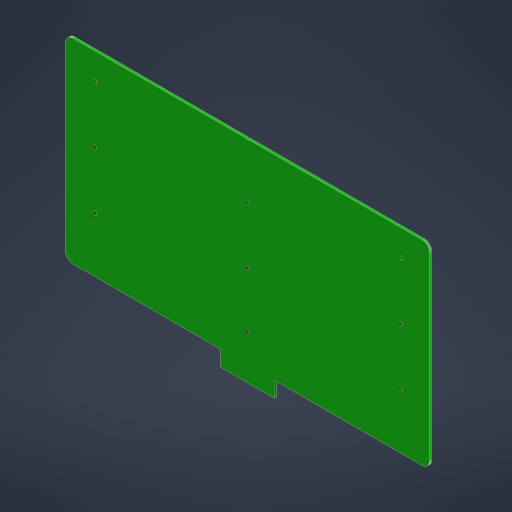
# Autodesk Inventor part: Platine_unten
Saved by Autodesk Inventor 2024.3 (Build 283343010, 343A)
## iProperties
Created: 2025-05-08
Part Number: Platine_unten
Material: Generisch
Document SubType Name: Modeling
Designer: David
Density: 1 g/cm^3
Appearance: Glatt - Schwarz
Author: David
Autodesk Inventor part; units mm, degrees
ref_plane "YZ Plane" through (0, 0, 0) normal (1, 0, 0) x (0, 1, 0)
ref_plane "XZ Plane" through (0, 0, 0) normal (0, 1, 0) x (-1, 0, 0)
ref_plane "XY Plane" through (0, 0, 0) normal (0, 0, 1) x (1, 0, 0)
sketch "Skizze1" plane through (0, 0, 0) normal (0, 1, 0) x (-1, 0, 0)
  line L0 (149.0026, -15.3777) -> (148.6057, -15.2961)
  line L1 (148.6057, -15.2961) -> (148.2026, -15.2551)
  line L2 (148.2026, -15.2551) -> (147.7974, -15.2551)
  line L3 (147.7974, -15.2551) -> (147.3943, -15.2961)
  line L4 (147.3943, -15.2961) -> (146.9974, -15.3777)
  line L5 (146.9974, -15.3777) -> (146.6108, -15.499)
  line L6 (146.6108, -15.499) -> (146.2384, -15.6588)
  line L7 (146.2384, -15.6588) -> (145.8841, -15.8554)
  line L8 (145.8841, -15.8554) -> (145.5516, -16.0869)
  line L9 (145.5516, -16.0869) -> (145.2441, -16.3508)
  line L10 (145.2441, -16.3508) -> (144.965, -16.6445)
  line L11 (144.965, -16.6445) -> (144.7169, -16.9649)
  line L12 (144.7169, -16.9649) -> (144.5026, -17.3088)
  line L13 (144.5026, -17.3088) -> (144.3242, -17.6726)
  line L14 (144.3242, -17.6726) -> (144.1834, -18.0525)
  line L15 (144.1834, -18.0525) -> (144.0819, -18.4448)
  line L16 (144.0819, -18.4448) -> (144.0205, -18.8453)
  line L17 (144.0205, -18.8453) -> (144, -19.25)
  line L18 (144, -19.25) -> (144, -20.5)
  line L19 (144, -20.5) -> (152, -20.5)
  line L20 (152, -20.5) -> (152, -19.25)
  line L21 (152, -19.25) -> (151.9795, -18.8453)
  line L22 (151.9795, -18.8453) -> (151.9181, -18.4448)
  line L23 (151.9181, -18.4448) -> (151.8166, -18.0525)
  line L24 (151.8166, -18.0525) -> (151.6758, -17.6726)
  line L25 (151.6758, -17.6726) -> (151.4974, -17.3088)
  line L26 (151.4974, -17.3088) -> (151.2831, -16.9649)
  line L27 (151.2831, -16.9649) -> (151.035, -16.6445)
  line L28 (151.035, -16.6445) -> (150.7559, -16.3508)
  line L29 (150.7559, -16.3508) -> (150.4484, -16.0869)
  line L30 (150.4484, -16.0869) -> (150.1159, -15.8554)
  line L31 (150.1159, -15.8554) -> (149.7616, -15.6588)
  line L32 (149.7616, -15.6588) -> (149.3892, -15.499)
  line L33 (149.3892, -15.499) -> (149.0026, -15.3777)
  line L34 (144, -20.5) -> (25, -20.5)
  line L35 (25, -20.5) -> (24.5642, -20.519)
  line L36 (24.5642, -20.519) -> (24.1318, -20.576)
  line L37 (24.1318, -20.576) -> (23.7059, -20.6704)
  line L38 (23.7059, -20.6704) -> (23.2899, -20.8015)
  line L39 (23.2899, -20.8015) -> (22.8869, -20.9685)
  line L40 (22.8869, -20.9685) -> (22.5, -21.1699)
  line L41 (22.5, -21.1699) -> (22.1321, -21.4042)
  line L42 (22.1321, -21.4042) -> (21.7861, -21.6698)
  line L43 (21.7861, -21.6698) -> (21.4645, -21.9645)
  line L44 (21.4645, -21.9645) -> (21.1698, -22.2861)
  line L45 (21.1698, -22.2861) -> (20.9042, -22.6321)
  line L46 (20.9042, -22.6321) -> (20.6699, -23)
  line L47 (20.6699, -23) -> (20.4685, -23.3869)
  line L48 (20.4685, -23.3869) -> (20.3015, -23.7899)
  line L49 (20.3015, -23.7899) -> (20.1704, -24.2059)
  line L50 (20.1704, -24.2059) -> (20.076, -24.6318)
  line L51 (20.076, -24.6318) -> (20.019, -25.0642)
  line L52 (20.019, -25.0642) -> (20, -25.5)
  line L53 (20, -25.5) -> (20, -153)
  line L54 (20, -153) -> (20.019, -153.4358)
  line L55 (20.019, -153.4358) -> (20.076, -153.8682)
  line L56 (20.076, -153.8682) -> (20.1704, -154.2941)
  line L57 (20.1704, -154.2941) -> (20.3015, -154.7101)
  line L58 (20.3015, -154.7101) -> (20.4685, -155.1131)
  line L59 (20.4685, -155.1131) -> (20.6699, -155.5)
  line L60 (20.6699, -155.5) -> (20.9042, -155.8679)
  line L61 (20.9042, -155.8679) -> (21.1698, -156.2139)
  line L62 (21.1698, -156.2139) -> (21.4645, -156.5355)
  line L63 (21.4645, -156.5355) -> (21.7861, -156.8302)
  line L64 (21.7861, -156.8302) -> (22.1321, -157.0958)
  line L65 (22.1321, -157.0958) -> (22.5, -157.3301)
  line L66 (22.5, -157.3301) -> (22.8869, -157.5315)
  line L67 (22.8869, -157.5315) -> (23.2899, -157.6985)
  line L68 (23.2899, -157.6985) -> (23.7059, -157.8296)
  line L69 (23.7059, -157.8296) -> (24.1318, -157.924)
  line L70 (24.1318, -157.924) -> (24.5642, -157.981)
  line L71 (24.5642, -157.981) -> (25, -158)
  line L72 (25, -158) -> (129, -158)
  line L73 (129, -158) -> (129, -169)
  line L74 (129, -169) -> (167, -169)
  line L75 (167, -169) -> (167, -158)
  line L76 (167, -158) -> (271, -158)
  line L77 (271, -158) -> (271.4358, -157.981)
  line L78 (271.4358, -157.981) -> (271.8682, -157.924)
  line L79 (271.8682, -157.924) -> (272.2941, -157.8296)
  line L80 (272.2941, -157.8296) -> (272.7101, -157.6985)
  line L81 (272.7101, -157.6985) -> (273.1131, -157.5315)
  line L82 (273.1131, -157.5315) -> (273.5, -157.3301)
  line L83 (273.5, -157.3301) -> (273.8679, -157.0958)
  line L84 (273.8679, -157.0958) -> (274.2139, -156.8302)
  line L85 (274.2139, -156.8302) -> (274.5355, -156.5355)
  line L86 (274.5355, -156.5355) -> (274.8302, -156.2139)
  line L87 (274.8302, -156.2139) -> (275.0958, -155.8679)
  line L88 (275.0958, -155.8679) -> (275.3301, -155.5)
  line L89 (275.3301, -155.5) -> (275.5315, -155.1131)
  line L90 (275.5315, -155.1131) -> (275.6985, -154.7101)
  line L91 (275.6985, -154.7101) -> (275.8296, -154.2941)
  line L92 (275.8296, -154.2941) -> (275.924, -153.8682)
  line L93 (275.924, -153.8682) -> (275.981, -153.4358)
  line L94 (275.981, -153.4358) -> (276, -153)
  line L95 (276, -153) -> (276, -25.5)
  line L96 (276, -25.5) -> (275.981, -25.0642)
  line L97 (275.981, -25.0642) -> (275.924, -24.6318)
  line L98 (275.924, -24.6318) -> (275.8296, -24.2059)
  line L99 (275.8296, -24.2059) -> (275.6985, -23.7899)
  line L100 (275.6985, -23.7899) -> (275.5315, -23.3869)
  line L101 (275.5315, -23.3869) -> (275.3301, -23)
  line L102 (275.3301, -23) -> (275.0958, -22.6321)
  line L103 (275.0958, -22.6321) -> (274.8302, -22.2861)
  line L104 (274.8302, -22.2861) -> (274.5355, -21.9645)
  line L105 (274.5355, -21.9645) -> (274.2139, -21.6698)
  line L106 (274.2139, -21.6698) -> (273.8679, -21.4042)
  line L107 (273.8679, -21.4042) -> (273.5, -21.1699)
  line L108 (273.5, -21.1699) -> (273.1131, -20.9685)
  line L109 (273.1131, -20.9685) -> (272.7101, -20.8015)
  line L110 (272.7101, -20.8015) -> (272.2941, -20.6704)
  line L111 (272.2941, -20.6704) -> (271.8682, -20.576)
  line L112 (271.8682, -20.576) -> (271.4358, -20.519)
  line L113 (271.4358, -20.519) -> (271, -20.5)
  line L114 (271, -20.5) -> (152, -20.5)
  line L115 (152, -20.5) -> (144, -20.5)
  line L116 (129, -169) -> (167, -169)
  line L117 (167, -169) -> (167, -158)
  line L118 (167, -158) -> (271, -158)
  line L119 (271, -158) -> (271.4358, -157.981)
  line L120 (271.4358, -157.981) -> (271.8682, -157.924)
  line L121 (271.8682, -157.924) -> (272.2941, -157.8296)
  line L122 (272.2941, -157.8296) -> (272.7101, -157.6985)
  line L123 (272.7101, -157.6985) -> (273.1131, -157.5315)
  line L124 (273.1131, -157.5315) -> (273.5, -157.3301)
  line L125 (273.5, -157.3301) -> (273.8679, -157.0958)
  line L126 (273.8679, -157.0958) -> (274.2139, -156.8302)
  line L127 (274.2139, -156.8302) -> (274.5355, -156.5355)
  line L128 (274.5355, -156.5355) -> (274.8302, -156.2139)
  line L129 (274.8302, -156.2139) -> (275.0958, -155.8679)
  line L130 (275.0958, -155.8679) -> (275.3301, -155.5)
  line L131 (275.3301, -155.5) -> (275.5315, -155.1131)
  line L132 (275.5315, -155.1131) -> (275.6985, -154.7101)
  line L133 (275.6985, -154.7101) -> (275.8296, -154.2941)
  line L134 (275.8296, -154.2941) -> (275.924, -153.8682)
  line L135 (275.924, -153.8682) -> (275.981, -153.4358)
  line L136 (275.981, -153.4358) -> (276, -153)
  line L137 (276, -153) -> (276, -25.5)
  line L138 (276, -25.5) -> (275.981, -25.0642)
  line L139 (275.981, -25.0642) -> (275.924, -24.6318)
  line L140 (275.924, -24.6318) -> (275.8296, -24.2059)
  line L141 (275.8296, -24.2059) -> (275.6985, -23.7899)
  line L142 (275.6985, -23.7899) -> (275.5315, -23.3869)
  line L143 (275.5315, -23.3869) -> (275.3301, -23)
  line L144 (275.3301, -23) -> (275.0958, -22.6321)
  line L145 (275.0958, -22.6321) -> (274.8302, -22.2861)
  line L146 (274.8302, -22.2861) -> (274.5355, -21.9645)
  line L147 (274.5355, -21.9645) -> (274.2139, -21.6698)
  line L148 (274.2139, -21.6698) -> (273.8679, -21.4042)
  line L149 (273.8679, -21.4042) -> (273.5, -21.1699)
  line L150 (273.5, -21.1699) -> (273.1131, -20.9685)
  line L151 (273.1131, -20.9685) -> (272.7101, -20.8015)
  line L152 (272.7101, -20.8015) -> (272.2941, -20.6704)
  line L153 (272.2941, -20.6704) -> (271.8682, -20.576)
  line L154 (271.8682, -20.576) -> (271.4358, -20.519)
  line L155 (271.4358, -20.519) -> (271, -20.5)
  line L156 (271, -20.5) -> (152, -20.5)
  line L157 (152, -20.5) -> (152, -19.25)
  line L158 (152, -19.25) -> (151.9795, -18.8453)
  line L159 (151.9795, -18.8453) -> (151.9181, -18.4448)
  line L160 (151.9181, -18.4448) -> (151.8166, -18.0525)
  line L161 (151.8166, -18.0525) -> (151.6758, -17.6726)
  line L162 (151.6758, -17.6726) -> (151.4974, -17.3088)
  line L163 (151.4974, -17.3088) -> (151.2831, -16.9649)
  line L164 (151.2831, -16.9649) -> (151.035, -16.6445)
  line L165 (151.035, -16.6445) -> (150.7559, -16.3508)
  line L166 (150.7559, -16.3508) -> (150.4484, -16.0869)
  line L167 (150.4484, -16.0869) -> (150.1159, -15.8554)
  line L168 (150.1159, -15.8554) -> (149.7616, -15.6588)
  line L169 (149.7616, -15.6588) -> (149.3892, -15.499)
  line L170 (149.3892, -15.499) -> (149.0026, -15.3777)
  line L171 (149.0026, -15.3777) -> (148.6057, -15.2961)
  line L172 (148.6057, -15.2961) -> (148.2026, -15.2551)
  line L173 (148.2026, -15.2551) -> (147.7974, -15.2551)
  line L174 (147.7974, -15.2551) -> (147.3943, -15.2961)
  line L175 (147.3943, -15.2961) -> (146.9974, -15.3777)
  line L176 (146.9974, -15.3777) -> (146.6108, -15.499)
  line L177 (146.6108, -15.499) -> (146.2384, -15.6588)
  line L178 (146.2384, -15.6588) -> (145.8841, -15.8554)
  line L179 (145.8841, -15.8554) -> (145.5516, -16.0869)
  line L180 (145.5516, -16.0869) -> (145.2441, -16.3508)
  line L181 (145.2441, -16.3508) -> (144.965, -16.6445)
  line L182 (144.965, -16.6445) -> (144.7169, -16.9649)
  line L183 (144.7169, -16.9649) -> (144.5026, -17.3088)
  line L184 (144.5026, -17.3088) -> (144.3242, -17.6726)
  line L185 (144.3242, -17.6726) -> (144.1834, -18.0525)
  line L186 (144.1834, -18.0525) -> (144.0819, -18.4448)
  line L187 (144.0819, -18.4448) -> (144.0205, -18.8453)
  line L188 (144.0205, -18.8453) -> (144, -19.25)
  line L189 (144, -19.25) -> (144, -20.5)
  line L190 (144, -20.5) -> (25, -20.5)
  line L191 (25, -20.5) -> (24.5642, -20.519)
  line L192 (24.5642, -20.519) -> (24.1318, -20.576)
  line L193 (24.1318, -20.576) -> (23.7059, -20.6704)
  line L194 (23.7059, -20.6704) -> (23.2899, -20.8015)
  line L195 (23.2899, -20.8015) -> (22.8869, -20.9685)
  line L196 (22.8869, -20.9685) -> (22.5, -21.1699)
  line L197 (22.5, -21.1699) -> (22.1321, -21.4042)
  line L198 (22.1321, -21.4042) -> (21.7861, -21.6698)
  line L199 (21.7861, -21.6698) -> (21.4645, -21.9645)
  line L200 (21.4645, -21.9645) -> (21.1698, -22.2861)
  line L201 (21.1698, -22.2861) -> (20.9042, -22.6321)
  line L202 (20.9042, -22.6321) -> (20.6699, -23)
  line L203 (20.6699, -23) -> (20.4685, -23.3869)
  line L204 (20.4685, -23.3869) -> (20.3015, -23.7899)
  line L205 (20.3015, -23.7899) -> (20.1704, -24.2059)
  line L206 (20.1704, -24.2059) -> (20.076, -24.6318)
  line L207 (20.076, -24.6318) -> (20.019, -25.0642)
  line L208 (20.019, -25.0642) -> (20, -25.5)
  line L209 (20, -25.5) -> (20, -153)
  line L210 (20, -153) -> (20.019, -153.4358)
  line L211 (20.019, -153.4358) -> (20.076, -153.8682)
  line L212 (20.076, -153.8682) -> (20.1704, -154.2941)
  line L213 (20.1704, -154.2941) -> (20.3015, -154.7101)
  line L214 (20.3015, -154.7101) -> (20.4685, -155.1131)
  line L215 (20.4685, -155.1131) -> (20.6699, -155.5)
  line L216 (20.6699, -155.5) -> (20.9042, -155.8679)
  line L217 (20.9042, -155.8679) -> (21.1698, -156.2139)
  line L218 (21.1698, -156.2139) -> (21.4645, -156.5355)
  line L219 (21.4645, -156.5355) -> (21.7861, -156.8302)
  line L220 (21.7861, -156.8302) -> (22.1321, -157.0958)
  line L221 (22.1321, -157.0958) -> (22.5, -157.3301)
  line L222 (22.5, -157.3301) -> (22.8869, -157.5315)
  line L223 (22.8869, -157.5315) -> (23.2899, -157.6985)
  line L224 (23.2899, -157.6985) -> (23.7059, -157.8296)
  line L225 (23.7059, -157.8296) -> (24.1318, -157.924)
  line L226 (24.1318, -157.924) -> (24.5642, -157.981)
  line L227 (24.5642, -157.981) -> (25, -158)
  line L228 (25, -158) -> (129, -158)
  line L229 (129, -158) -> (129, -169)
  line L230 (137.25, -162.4) -> (137.25, -165.9)
  line L231 (137.25, -165.9) -> (158.75, -165.9)
  line L232 (158.75, -165.9) -> (137.25, -165.9)
  line L233 (137.25, -165.9) -> (158.75, -165.9)
  line L234 (158.75, -165.9) -> (158.75, -162.4)
  line L235 (158.75, -162.4) -> (137.25, -162.4)
  line L236 (137.75, -162.9) -> (140.25, -162.9)
  line L237 (140.25, -162.9) -> (140.25, -165.4)
  line L238 (140.25, -165.4) -> (137.75, -165.4)
  line L239 (137.75, -165.4) -> (137.75, -162.9)
  line L240 (140.75, -162.9) -> (143.25, -162.9)
  line L241 (143.25, -162.9) -> (143.25, -165.4)
  line L242 (143.25, -165.4) -> (140.75, -165.4)
  line L243 (140.75, -165.4) -> (140.75, -162.9)
  line L244 (143.75, -162.9) -> (146.25, -162.9)
  line L245 (146.25, -162.9) -> (146.25, -165.4)
  line L246 (146.25, -165.4) -> (143.75, -165.4)
  line L247 (143.75, -165.4) -> (143.75, -162.9)
  line L248 (146.75, -162.9) -> (149.25, -162.9)
  line L249 (149.25, -162.9) -> (149.25, -165.4)
  line L250 (149.25, -165.4) -> (146.75, -165.4)
  line L251 (146.75, -165.4) -> (146.75, -162.9)
  line L252 (149.75, -162.9) -> (152.25, -162.9)
  line L253 (152.25, -162.9) -> (152.25, -165.4)
  line L254 (152.25, -165.4) -> (149.75, -165.4)
  line L255 (149.75, -165.4) -> (149.75, -162.9)
  line L256 (152.75, -162.9) -> (155.25, -162.9)
  line L257 (155.25, -162.9) -> (155.25, -165.4)
  line L258 (155.25, -165.4) -> (152.75, -165.4)
  line L259 (152.75, -165.4) -> (152.75, -162.9)
  line L260 (155.75, -162.9) -> (158.25, -162.9)
  line L261 (158.25, -162.9) -> (158.25, -165.4)
  line L262 (158.25, -165.4) -> (155.75, -165.4)
  line L263 (155.75, -165.4) -> (155.75, -162.9)
  line L264 (129, -169) -> (129, -158)
  line L265 (129, -158) -> (25, -158)
  line L266 (25, -158) -> (24.5642, -157.981)
  line L267 (24.5642, -157.981) -> (24.1318, -157.924)
  line L268 (24.1318, -157.924) -> (23.7059, -157.8296)
  line L269 (23.7059, -157.8296) -> (23.2899, -157.6985)
  line L270 (23.2899, -157.6985) -> (22.8869, -157.5315)
  line L271 (22.8869, -157.5315) -> (22.5, -157.3301)
  line L272 (22.5, -157.3301) -> (22.1321, -157.0958)
  line L273 (22.1321, -157.0958) -> (21.7861, -156.8302)
  line L274 (21.7861, -156.8302) -> (21.4645, -156.5355)
  line L275 (21.4645, -156.5355) -> (21.1698, -156.2139)
  line L276 (21.1698, -156.2139) -> (20.9042, -155.8679)
  line L277 (20.9042, -155.8679) -> (20.6699, -155.5)
  line L278 (20.6699, -155.5) -> (20.4685, -155.1131)
  line L279 (20.4685, -155.1131) -> (20.3015, -154.7101)
  line L280 (20.3015, -154.7101) -> (20.1704, -154.2941)
  line L281 (20.1704, -154.2941) -> (20.076, -153.8682)
  line L282 (20.076, -153.8682) -> (20.019, -153.4358)
  line L283 (20.019, -153.4358) -> (20, -153)
  line L284 (20, -153) -> (20, -25.5)
  line L285 (20, -25.5) -> (20.019, -25.0642)
  line L286 (20.019, -25.0642) -> (20.076, -24.6318)
  line L287 (20.076, -24.6318) -> (20.1704, -24.2059)
  line L288 (20.1704, -24.2059) -> (20.3015, -23.7899)
  line L289 (20.3015, -23.7899) -> (20.4685, -23.3869)
  line L290 (20.4685, -23.3869) -> (20.6699, -23)
  line L291 (20.6699, -23) -> (20.9042, -22.6321)
  line L292 (20.9042, -22.6321) -> (21.1698, -22.2861)
  line L293 (21.1698, -22.2861) -> (21.4645, -21.9645)
  line L294 (21.4645, -21.9645) -> (21.7861, -21.6698)
  line L295 (21.7861, -21.6698) -> (22.1321, -21.4042)
  line L296 (22.1321, -21.4042) -> (22.5, -21.1699)
  line L297 (22.5, -21.1699) -> (22.8869, -20.9685)
  line L298 (22.8869, -20.9685) -> (23.2899, -20.8015)
  line L299 (23.2899, -20.8015) -> (23.7059, -20.6704)
  line L300 (23.7059, -20.6704) -> (24.1318, -20.576)
  line L301 (24.1318, -20.576) -> (24.5642, -20.519)
  line L302 (24.5642, -20.519) -> (25, -20.5)
  line L303 (25, -20.5) -> (144, -20.5)
  line L304 (144, -20.5) -> (144, -19.25)
  line L305 (144, -19.25) -> (144.0205, -18.8453)
  line L306 (144.0205, -18.8453) -> (144.0819, -18.4448)
  line L307 (144.0819, -18.4448) -> (144.1834, -18.0525)
  line L308 (144.1834, -18.0525) -> (144.3242, -17.6726)
  line L309 (144.3242, -17.6726) -> (144.5026, -17.3088)
  line L310 (144.5026, -17.3088) -> (144.7169, -16.9649)
  line L311 (144.7169, -16.9649) -> (144.965, -16.6445)
  line L312 (144.965, -16.6445) -> (145.2441, -16.3508)
  line L313 (145.2441, -16.3508) -> (145.5516, -16.0869)
  line L314 (145.5516, -16.0869) -> (145.8841, -15.8554)
  line L315 (145.8841, -15.8554) -> (146.2384, -15.6588)
  line L316 (146.2384, -15.6588) -> (146.6108, -15.499)
  line L317 (146.6108, -15.499) -> (146.9974, -15.3777)
  line L318 (146.9974, -15.3777) -> (147.3943, -15.2961)
  line L319 (147.3943, -15.2961) -> (147.7974, -15.2551)
  line L320 (147.7974, -15.2551) -> (148.2026, -15.2551)
  line L321 (148.2026, -15.2551) -> (148.6057, -15.2961)
  line L322 (148.6057, -15.2961) -> (149.0026, -15.3777)
  line L323 (149.0026, -15.3777) -> (149.3892, -15.499)
  line L324 (149.3892, -15.499) -> (149.7616, -15.6588)
  line L325 (149.7616, -15.6588) -> (150.1159, -15.8554)
  line L326 (150.1159, -15.8554) -> (150.4484, -16.0869)
  line L327 (150.4484, -16.0869) -> (150.7559, -16.3508)
  line L328 (150.7559, -16.3508) -> (151.035, -16.6445)
  line L329 (151.035, -16.6445) -> (151.2831, -16.9649)
  line L330 (151.2831, -16.9649) -> (151.4974, -17.3088)
  line L331 (151.4974, -17.3088) -> (151.6758, -17.6726)
  line L332 (151.6758, -17.6726) -> (151.8166, -18.0525)
  line L333 (151.8166, -18.0525) -> (151.9181, -18.4448)
  line L334 (151.9181, -18.4448) -> (151.9795, -18.8453)
  line L335 (151.9795, -18.8453) -> (152, -19.25)
  line L336 (152, -19.25) -> (152, -20.5)
  line L337 (152, -20.5) -> (271, -20.5)
  line L338 (271, -20.5) -> (271.4358, -20.519)
  line L339 (271.4358, -20.519) -> (271.8682, -20.576)
  line L340 (271.8682, -20.576) -> (272.2941, -20.6704)
  line L341 (272.2941, -20.6704) -> (272.7101, -20.8015)
  line L342 (272.7101, -20.8015) -> (273.1131, -20.9685)
  line L343 (273.1131, -20.9685) -> (273.5, -21.1699)
  line L344 (273.5, -21.1699) -> (273.8679, -21.4042)
  line L345 (273.8679, -21.4042) -> (274.2139, -21.6698)
  line L346 (274.2139, -21.6698) -> (274.5355, -21.9645)
  line L347 (274.5355, -21.9645) -> (274.8302, -22.2861)
  line L348 (274.8302, -22.2861) -> (275.0958, -22.6321)
  line L349 (275.0958, -22.6321) -> (275.3301, -23)
  line L350 (275.3301, -23) -> (275.5315, -23.3869)
  line L351 (275.5315, -23.3869) -> (275.6985, -23.7899)
  line L352 (275.6985, -23.7899) -> (275.8296, -24.2059)
  line L353 (275.8296, -24.2059) -> (275.924, -24.6318)
  line L354 (275.924, -24.6318) -> (275.981, -25.0642)
  line L355 (275.981, -25.0642) -> (276, -25.5)
  line L356 (276, -25.5) -> (276, -153)
  line L357 (276, -153) -> (275.981, -153.4358)
  line L358 (275.981, -153.4358) -> (275.924, -153.8682)
  line L359 (275.924, -153.8682) -> (275.8296, -154.2941)
  line L360 (275.8296, -154.2941) -> (275.6985, -154.7101)
  line L361 (275.6985, -154.7101) -> (275.5315, -155.1131)
  line L362 (275.5315, -155.1131) -> (275.3301, -155.5)
  line L363 (275.3301, -155.5) -> (275.0958, -155.8679)
  line L364 (275.0958, -155.8679) -> (274.8302, -156.2139)
  line L365 (274.8302, -156.2139) -> (274.5355, -156.5355)
  line L366 (274.5355, -156.5355) -> (274.2139, -156.8302)
  line L367 (274.2139, -156.8302) -> (273.8679, -157.0958)
  line L368 (273.8679, -157.0958) -> (273.5, -157.3301)
  line L369 (273.5, -157.3301) -> (273.1131, -157.5315)
  line L370 (273.1131, -157.5315) -> (272.7101, -157.6985)
  line L371 (272.7101, -157.6985) -> (272.2941, -157.8296)
  line L372 (272.2941, -157.8296) -> (271.8682, -157.924)
  line L373 (271.8682, -157.924) -> (271.4358, -157.981)
  line L374 (271.4358, -157.981) -> (271, -158)
  line L375 (271, -158) -> (167, -158)
  line L376 (167, -158) -> (167, -169)
  line L377 (146.7, -165.9) -> (146.7, -167.1)
  line L378 (146.7, -167.1) -> (149.3, -167.1)
  line L379 (149.3, -167.1) -> (149.3, -165.9)
  circle A0 centre (255.5, -119.25) radius 1.6
  circle A1 centre (148, -138) radius 1.6
  circle A2 centre (255.5, -79.25) radius 1.6
  circle A3 centre (148, -99.25) radius 1.6
  circle A4 centre (40.5, -119.25) radius 1.6
  circle A5 centre (40.5, -79.25) radius 1.6
  circle A6 centre (148, -59.25) radius 1.6
  circle A7 centre (255.5, -39.25) radius 1.6
  circle A8 centre (148, -19.25) radius 1.6
  circle A9 centre (40.5, -39.25) radius 1.6
  point P0 (0, 0)
  point P1 (148.9987, -20.5)
  point P2 (147.0013, -20.5)
  point P3 (276, -25.5)
  constraints: 760 end point, 10 centre point
extrude "Extrusion1" add sketch "Skizze1" against normal blind 1.6 contours L114 L113 L112 L111 L110 L109 L108 L107 L106 L105 L104 L103 L102 L101 L100 L99 L98 L97 L96 L95 L94 L93 L92 L91 L90 L89 L88 L87 L86 L85 L84 L83 L82 L81 L80 L79 L78 L77 L76 L75 L74 L73 L72 L71 L70 L69 L68 L67 L66 L65 L64 L63 L62 L61 L60 L59 L58 L57 L56 L55 L54 L53 L52 L51 L50 L49 L48 L47 L46 L45 L44 L43 L42 L41 L40 L39 L38 L37 L36 L35 L34 L19 A8 | L235 L234 L231 L230 | L231 L379 L378 L377 | L236 L237 L238 L239 | L240 L241 L242 L243 | L244 L245 L246 L247 | L248 L249 L250 L251 | L252 L253 L254 L255 | L256 L257 L258 L259 | L260 L261 L262 L263
extrude "Extrusion2" add sketch "Skizze1" along normal blind 10.4 contours L235 L234 L231 L230 | L231 L379 L378 L377
extrude "Extrusion3" cut sketch "Skizze1" along normal blind 8 contours L231 L379 L378 L377
chamfer "Fasen1" distance 1.2 angle 45 1 edges at (-148, 10.4, -167.1)
